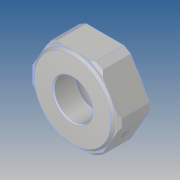
# Autodesk Inventor part: support_canon
Saved by Autodesk Inventor 2019 (Build 230136000, 136)
## iProperties
Created: 2019-03-26
Part Number: support_canon
Material: Aluminium 6061
Document SubType Name: Modeling
Designer: theor
Density: 2.7 g/cm^3
Appearance: Aluminium - Plat
Mass: 29.353 g
Surface Area: 41.7023 cm^2
Volume: 10.8715 cm^3
Author: theor
Autodesk Inventor part; units mm, degrees
note: some values were not read from the file. Chosen so that the rebuilt part matches the saved one: sketch regions of "Extrusion1"; pattern direction of "Réseau circulaire2".
ref_plane "YZ Plane" through (0, 0, 0) normal (1, 0, 0) x (0, 1, 0)
ref_plane "XZ Plane" through (0, 0, 0) normal (0, 1, 0) x (-1, 0, 0)
sketch "Esquisse1" plane through (0, 0, 0) normal (1, 0, 0) x (0, 1, 0)
  line L0 (0, 0) -> (0, 17.727)
  line L1 (8.25, 5) -> (8.25, 15)
  line L2 (8.25, 5) -> (11, 5)
  line L3 (11, 5) -> (11, 0)
  line L4 (17.5, 14) -> (17.5, 1)
  line L5 (16.5, 0) -> (11, 0)
  line L6 (8.25, 15) -> (16.5, 15)
  line L7 (16.5, 15) -> (17.5, 14)
  line L8 (17.5, 1) -> (16.5, 0)
  dimension "d1" = 16.5
  dimension "d2" = 22
  dimension "d3" = 35
  dimension "d4" = 5
  dimension "d71" = 1
  dimension "d72" = 1
  dimension "d77" = 1
  dimension "d78" = 1
  dimension "d82" = 15
  constraints: 18 end point, 4 vertical, 3 horizontal, 1 horizontal alignment
  measures "d1" diameter of L1 L0
  measures "d2" diameter of L3 L0
  measures "d3" diameter of L4 L0
  measures "d4" distance of L2.end L3.end
  measures "d71" horizontal distance of L4.end L5.start
  measures "d72" horizontal distance of L4.end L5.start
  measures "d77" horizontal distance of L6.end L4.start
  measures "d78" horizontal distance of L6.end L4.start
  measures "d82" distance between parallel lines of L6 L5
revolve "Révolution1" add sketch "Esquisse1" angle 360 about axis through (0, 0, 0) along (0, 0, 1)
ref_plane "Plan de construction1" through (0, 0, 1) normal (0, 0, -1) x (-1, 0, 0)
sketch "Esquisse2" plane through (0, 0, 1) normal (0, 0, -1) x (-1, 0, 0)
  line L0 (10.1036, 17.5) -> (20.2073, 0)
  line L1 (20.2073, 0) -> (10.1036, -17.5)
  line L2 (10.1036, -17.5) -> (-10.1036, -17.5)
  line L3 (-10.1036, -17.5) -> (-20.2073, 0)
  line L4 (-20.2073, 0) -> (-10.1036, 17.5)
  line L5 (-10.1036, 17.5) -> (10.1036, 17.5)
  circle A0 centre (0, 0) radius 17.5 projected
  arc A1 (-15.1554, 8.75) -> (15.1554, 8.75) centre (0, 0) ccw
  constraints: 12 end point, 4 point on circle, 2 coincident, 2 midpoint, 1 centre point, 1 horizontal, 1 tangent, 13 other
extrude "Extrusion1" add sketch "Esquisse2" against normal blind 13 contours L0 A0 L5 | L0 L1 A0 | A0 L4 L5 | A0 L3 L4 | L1 L2 A0 | A0 L2 L3
chamfer "Chanfrein1" distance 0.5 angle 45 2 edges at (0, -11, 0) (0, -11, 5)
chamfer "Chanfrein2" distance 2 angle 45 6 edges at (10.1036, 17.5, 7.5) (20.2073, 0, 7.5) (10.1036, -17.5, 7.5) (-10.1036, -17.5, 7.5) (-20.2073, 0, 7.5) (-10.1036, 17.5, 7.5)
sketch "Esquisse3" plane through (-8.1036, -17.5, 1) normal (0, -1, 0) x (1, 0, 0)
  line L0 (0, 13) -> (16.2073, 13) projected
  line L1 (-8.3964, -1) -> (24.6036, -1) projected
  line L2 (0, 0) -> (0, 13) projected
  point P0 (8.1036, -1)
  point P1 (8.1036, 6.5)
  point P2 (8.1036, 0)
  point P3 (16.2073, 0)
  point P4 (8.1036, 0)
  point P5 (8.1036, 13)
  point P6 (0, 6.5)
  constraints: 1 horizontal alignment, 1 midpoint, 1 vertical alignment
hole "Perçage1" at (0, -17.5, 7.5) direction (0, 1, 0) diameter 3.242 depth 6 tip angle 118 thread size "M4x0.7" class "6H" standard "ISO Metric profile"
chamfer "Chanfrein4" distance 0.5 angle 45 2 edges at (0, -8.25, 15) (0, -8.25, 5)
chamfer "Chanfrein5" distance 1 angle 45 6 edges at (9.6036, 16.634, 14) (19.2073, 0, 14) (9.6036, -16.634, 14) (-9.6036, -16.634, 14) (-19.2073, 0, 14) (-9.6036, 16.634, 14)
pattern_circular "Réseau circulaire2" count 3 over 120 about axis through (0, 0, -10) along (0, 0, 1) of "Perçage1" both ways yes
equation "\"d72\" = d71"
equation "\"d78\" = d77"
